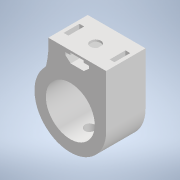
# Autodesk Inventor part: MotorBearingHolder
Saved by Autodesk Inventor 2020.2 (Build 242310000, 310)
## iProperties
Created: 2020-01-14
Part Number: MotorBearingHolder
Material: Generic
Document SubType Name: Modeling
Designer: yukin
Density: 1 g/cm^3
Appearance: Default
Author: yukin
Autodesk Inventor part; units mm, degrees
ref_plane "YZ Plane" through (0, 0, 0) normal (1, 0, 0) x (0, 1, 0)
sketch "Sketch1" plane through (0, 0, 0) normal (0, 0, 1) x (1, 0, 0)
  line L0 (-13.97, -12.7) -> (13.97, -12.7)
  line L1 (13.97, -12.7) -> (13.97, 12.7)
  line L2 (13.97, 12.7) -> (-13.97, 12.7)
  line L3 (-13.97, 12.7) -> (-13.97, -12.7)
  line L4 (-13.97, -12.7) -> (13.97, 12.7) construction
  line L5 (13.97, -12.7) -> (-13.97, 12.7) construction
  arc A0 (-13.97, -12.7) -> (13.97, -12.7) centre (0, -12.7) ccw
  circle A1 centre (-3.3455, -12.7) radius 11.811
  line L6 (0, -12.7) -> (-13.97, -12.7)
  line L7 (0, -12.7) -> (-6.985, -12.7)
  circle A2 centre (-3.3455, -12.7) radius 17.3155
  arc A3 (-20.6609, -12.7) -> (-13.97, 12.7) centre (-56.001, 10.1906) ccw
  point P0 (0, 0)
  point P1 (-15.1565, -0.038)
  dimension "d0" = 27.94
  dimension "d1" = 25.4
  dimension "d2" = 23.622
  constraints: 16 end point, 6 point on circle, 4 centre point, 3 midpoint, 2 parallel, 2 tangent, 1 coincident, 1 horizontal, 1 perpendicular
  measures "d0" distance of L1.end L2.end
  measures "d1" distance of L0.end L1.end
  measures "d2" diameter of A1
sketch "Sketch5" plane through (0, 0, 0) normal (0, 0, 1) x (1, 0, 0)
  line L0 (0, 12.7) -> (0, 6.35)
  line L1 (0, 12.7) -> (0, 9.525)
  line L2 (5.715, 7.3025) -> (-5.715, 7.3025)
  line L3 (-5.715, 7.3025) -> (-5.715, 11.7475)
  line L4 (-5.715, 11.7475) -> (5.715, 11.7475)
  line L5 (5.715, 11.7475) -> (5.715, 7.3025)
  line L6 (5.715, 7.3025) -> (-5.715, 11.7475) construction
  line L7 (-5.715, 7.3025) -> (5.715, 11.7475) construction
  line L8 (5.715, 11.7475) -> (3.175, 11.7475)
  line L9 (3.175, 11.7475) -> (3.175, 10.7597)
  line L10 (3.175, 10.7597) -> (5.715, 10.7597)
  line L11 (5.715, 10.7597) -> (5.715, 11.7475)
  line L12 (-5.715, 11.7475) -> (-3.2581, 11.7475)
  line L13 (-3.2581, 11.7475) -> (-3.2581, 10.792)
  line L14 (-3.2581, 10.792) -> (-5.715, 10.792)
  line L15 (-5.715, 10.792) -> (-5.715, 11.7475)
  line L16 (5.715, 9.525) -> (3.175, 7.3025)
  line L17 (-5.715, 9.525) -> (-3.175, 7.3025)
  point P0 (0, 0)
  point P1 (5.715, 10.7597)
  point P2 (-3.2581, 11.7475)
  point P3 (-5.715, 10.792)
  dimension "d5" = 4.445
  dimension "d6" = 11.43
  dimension "d7" = 2.54
  constraints: 36 end point, 6 parallel, 5 midpoint, 4 point on line, 3 horizontal, 3 perpendicular
  measures "d5" distance of L2.end L3.end
  measures "d6" distance of L2.start L2.end
  measures "d7" distance of L10.end L9.end
ref_plane "Work Plane4" through (-13.97, 12.7, 0) normal (0, 1, 0) x (1, 0, 0)
sketch "Sketch6" plane through (-13.97, 12.7, 0) normal (0, 1, 0) x (1, 0, 0)
  circle A0 centre (13.5492, -9.5343) radius 2.54
  dimension "d19" = 5.08
  constraints: 1 centre point
  measures "d19" diameter of A0
extrude "Extrusion7" add sketch "Sketch1" along normal blind 19.05 contours A1 A0 A2 A3 L3 | L3 A2 L0 A1 | A1 L0 A0 | A2 A3 L3 | L3 A3 L2 L1 A2 | A3 A2 picked at (12.0052, -13.7923)
extrude "Extrusion8" cut sketch "Sketch5" along normal blind 20.32 contours L4 L9 L10 L5 L16 L2 L0 | L0 L2 L17 L3 L14 L13 L4
extrude "Extrusion9" cut sketch "Sketch6" against normal blind 15.24
fillet "Fillet1" radius 3.175 1 edges at (-15.1565, -0.038, 9.525)
sketch "Sketch10" plane through (-13.97, 12.7, 0) normal (0, 1, 0) x (1, 0, 0)
  line L0 (13.97, 0) -> (13.97, -20.32)
  line L1 (0.0748, -19.05) -> (0.0748, 0) projected
  line L2 (0.0748, -9.525) -> (27.94, -9.525)
  line L3 (27.94, 0) -> (27.94, -19.05) projected
  line L4 (3.9773, -13.335) -> (1.6913, -13.335)
  line L5 (1.6913, -13.335) -> (1.6913, -5.715)
  line L6 (1.6913, -5.715) -> (3.9773, -5.715)
  line L7 (3.9773, -5.715) -> (3.9773, -13.335)
  line L8 (3.9773, -13.335) -> (1.6913, -5.715) construction
  line L9 (1.6913, -13.335) -> (3.9773, -5.715) construction
  line L10 (23.9627, -13.335) -> (26.2487, -13.335)
  line L11 (26.2487, -13.335) -> (26.2487, -5.715)
  line L12 (26.2487, -5.715) -> (23.9627, -5.715)
  line L13 (23.9627, -5.715) -> (23.9627, -13.335)
  point P0 (2.8343, -9.525)
  dimension "d32" = 2.286
  dimension "d33" = 7.62
  constraints: 24 end point, 4 midpoint, 4 symmetric about line, 2 parallel, 1 horizontal, 1 perpendicular, 1 point on line
  measures "d32" distance of L5.end L6.end
  measures "d33" distance of L6.end L4.start
extrude "Extrusion10" cut sketch "Sketch10" against normal blind 2.54
ref_plane "Work Plane5" through (-3.3455, -30.0155, 0) normal (0, 1, 0) x (-1, 0, 0)
sketch "Sketch11" plane through (-3.3455, -30.0155, 0) normal (0, 1, 0) x (-1, 0, 0)
  line L0 (-0.1705, 0) -> (-0.1705, 19.05) projected
  circle A0 centre (-0.1705, 9.525) radius 2.54
  point P0 (-3.3455, 0)
  dimension "d36" = 5.08
  constraints: 1 centre point, 1 midpoint
  measures "d36" diameter of A0
extrude "Extrusion11" cut sketch "Sketch11" along normal blind 15.24
body "Solid2"
